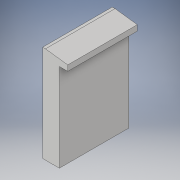
# Autodesk Inventor part: straightrib
Saved by Autodesk Inventor 2019 (Build 230136000, 136)
## iProperties
Created: 2019-01-18
Part Number: straightrib
Material: Generic
Document SubType Name: Modeling
Designer: assman
Density: 1 g/cm^3
Appearance: Default
Author: assman
Autodesk Inventor part; units mm, degrees
ref_plane "YZ Plane" through (0, 0, 0) normal (1, 0, 0) x (0, 1, 0)
ref_plane "XZ Plane" through (0, 0, 0) normal (0, 1, 0) x (-1, 0, 0)
ref_plane "XY Plane" through (0, 0, 0) normal (0, 0, 1) x (1, 0, 0)
sketch "Sketch1" plane through (0, 0, 0) normal (0, 1, 0) x (-1, 0, 0)
  line L0 (-1.2, -5) -> (1.2, -5)
  line L1 (1.2, -5) -> (1.2, 5)
  line L2 (1.2, 5) -> (-1.2, 5)
  line L3 (-1.2, 5) -> (-1.2, -5)
  line L4 (-1.2, -5) -> (1.2, 5) construction
  line L5 (1.2, -5) -> (-1.2, 5) construction
  point P0 (0, 0)
  dimension "length" = 10
  dimension "width" = 2.4
  constraints: 12 end point, 2 midpoint, 2 parallel, 1 horizontal, 1 perpendicular
  measures "length" distance of L0.end L1.end
  measures "width" distance of L1.end L2.end
extrude "Extrusion1" add sketch "Sketch1" along normal blind 12.65
sketch "Sketch3" plane through (-1.2, 0, 5) normal (0, 0, 1) x (1, 0, 0)
  line L0 (2.4, 12.65) -> (3.6, 12.65)
  line L1 (3.6, 12.65) -> (3.6, 13.45)
  line L2 (0, 13.85) -> (0.4, 13.85)
  line L3 (3.6, 13.45) -> (0.4, 13.85)
  line L4 (0, 13.85) -> (0, 12.65)
  line L5 (2.4, 12.65) -> (0, 12.65) projected
  line L6 (0, 12.65) -> (2.4, 12.65)
  line L7 (0, 0) -> (0, 12.65) projected
  line L8 (2.4, 0) -> (2.4, 12.65) projected
  point P0 (1.2, 0)
  dimension "fixer" = 1.2
  dimension "d8" = 0.8
  dimension "d11" = 0.4
  dimension "d12" = 1.2
  constraints: 12 end point, 3 perpendicular, 1 collinear
  measures "fixer" distance of L0.start L0.end
  measures "d8" distance of L0.end L1.end
  measures "d11" distance of L2.start L2.end
  measures "d12" distance of L2.start L4.end
extrude "Extrusion2" add sketch "Sketch3" against normal blind 10
equation "\"d6\" = length"
equation "\"TOL\" = 0.15"
body "Solid1"
